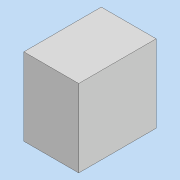
# Autodesk Inventor part: Frame generator
Saved by Autodesk Inventor 2020 (Build 240168000, 168)
## iProperties
Created: 2020-04-09
Part Number: Frame generator
Material: Generic
Document SubType Name: Modeling
Designer: Simon
Density: 1 g/cm^3
Appearance: Default
Author: Simon
Autodesk Inventor part; units mm, degrees
ref_plane "YZ Plane" through (0, 0, 0) normal (1, 0, 0) x (0, 1, 0)
ref_plane "XZ Plane" through (0, 0, 0) normal (0, 1, 0) x (-1, 0, 0)
ref_plane "XY Plane" through (0, 0, 0) normal (0, 0, 1) x (1, 0, 0)
sketch "Sketch1" plane through (0, 0, 0) normal (0, 0, 1) x (1, 0, 0)
  line L0 (-85.25, -120.25) -> (85.25, -120.25)
  line L1 (85.25, -120.25) -> (85.25, 120.25)
  line L2 (85.25, 120.25) -> (-85.25, 120.25)
  line L3 (-85.25, 120.25) -> (-85.25, -120.25)
  line L4 (-85.25, -120.25) -> (85.25, 120.25) construction
  line L5 (85.25, -120.25) -> (-85.25, 120.25) construction
  point P0 (0, 0)
  dimension "d0" = 170.5
  dimension "d1" = 240.5
  constraints: 12 end point, 2 midpoint, 2 parallel, 1 horizontal, 1 perpendicular
  measures "d0" distance of L2.end L1.end
  measures "d1" distance of L1.end L0.end
extrude "Extrusion1" add sketch "Sketch1" along normal mid plane 240.5
body "Solid1"
